Autodesk Inventor part; units mm, degrees
(part 3 of 5)
  line L374 (16.7292, 18.0861) -> (16.8663, 18.4528)
  line L375 (16.8663, 18.4528) -> (16.7213, 18.5673)
  arc A972 (16.7213, 18.5673) -> (16.5062, 18.7273) centre (13.8338, 14.9109) ccw
  arc A973 (16.5062, 18.7273) -> (16.4174, 18.7432) centre (16.4446, 18.6392) ccw
  arc A974 (16.4174, 18.7432) -> (16.3499, 18.6856) centre (16.4431, 18.6448) ccw
  arc A975 (16.3499, 18.6856) -> (16.2535, 18.445) centre (20.1386, 17.0284) ccw
  arc A976 (7.6941, 18.0877) -> (7.7913, 18.19) centre (6.7179, 19.1135) ccw
  arc A977 (7.5704, 17.9771) -> (7.6941, 18.0877) centre (5.8408, 20.0352) ccw
  arc A978 (7.4412, 17.8752) -> (7.5704, 17.9771) centre (5.8587, 20.0139) ccw
  arc A979 (7.3271, 17.7998) -> (7.4412, 17.8752) centre (6.68, 18.9039) ccw
  arc A980 (7.3271, 17.7998) -> (7.1576, 17.6869) centre (8.2213, 16.2738) ccw
  arc A981 (7.1576, 17.6869) -> (7.1147, 17.6052) centre (7.2224, 17.6008) ccw
  arc A982 (7.1147, 17.6052) -> (7.1453, 17.5068) centre (7.2684, 17.599) ccw
  arc A983 (7.1453, 17.5068) -> (7.307, 17.3046) centre (10.3922, 19.9382) ccw
  arc A984 (7.307, 17.3046) -> (7.3807, 17.2275) centre (8.0311, 17.9227) ccw
  arc A985 (7.3807, 17.2275) -> (7.4351, 17.1973) centre (7.468, 17.3209) ccw
  arc A986 (7.4351, 17.1973) -> (7.4946, 17.1979) centre (7.4638, 17.3048) ccw
  arc A987 (7.4946, 17.1979) -> (7.5838, 17.2309) centre (7.3149, 17.821) ccw
  arc A988 (7.5838, 17.2309) -> (7.7872, 17.3447) centre (6.9978, 18.5171) ccw
  arc A989 (7.7872, 17.3447) -> (7.9869, 17.499) centre (6.7051, 18.9518) ccw
  arc A990 (7.9869, 17.499) -> (8.1701, 17.6827) centre (6.6366, 19.0294) ccw
  arc A991 (8.1701, 17.6827) -> (8.3244, 17.8844) centre (6.7621, 18.9192) ccw
  arc A992 (8.3244, 17.8844) -> (8.3941, 17.9924) centre (3.8751, 20.8314) ccw
  arc A993 (8.3941, 17.9924) -> (8.4528, 18.0896) centre (5.6287, 19.7297) ccw
  arc A994 (8.4528, 18.0896) -> (8.4998, 18.1724) centre (4.4364, 20.4221) ccw
  arc A995 (8.4998, 18.1724) -> (8.5063, 18.1976) centre (8.4543, 18.1976) ccw
  arc A996 (8.5063, 18.1976) -> (8.4823, 18.2379) centre (8.4603, 18.1976) ccw
  arc A997 (8.4823, 18.2379) -> (8.2984, 18.3345) centre (5.3457, 12.4849) ccw
  arc A998 (8.2984, 18.3345) -> (8.1156, 18.4216) centre (6.279, 14.3339) ccw
  arc A999 (8.1156, 18.4216) -> (8.0392, 18.4333) centre (8.0563, 18.2894) ccw
  arc A1000 (8.0392, 18.4333) -> (8.014, 18.4217) centre (8.0445, 18.3884) ccw
  arc A1001 (8.014, 18.4217) -> (7.9487, 18.3598) centre (9.8459, 16.4267) ccw
  arc A1002 (7.9487, 18.3598) -> (7.873, 18.2817) centre (9.4826, 16.7968) ccw
  arc A1003 (7.873, 18.2817) -> (7.7913, 18.19) centre (10.4757, 15.8807) ccw
  line L376 (9.6608, 18.2942) -> (9.4652, 18.1559)
  line L377 (9.4652, 18.1559) -> (9.5952, 17.9907)
  arc A1004 (9.5952, 17.9907) -> (9.6704, 17.9062) centre (10.3274, 18.5667) ccw
  arc A1005 (9.6704, 17.9062) -> (9.8032, 17.7781) centre (13.9276, 22.186) ccw
  arc A1006 (9.8032, 17.7781) -> (9.9598, 17.6361) centre (14.449, 22.7432) ccw
  arc A1007 (9.9598, 17.6361) -> (10.1207, 17.499) centre (14.4559, 22.751) ccw
  line L378 (10.1207, 17.499) -> (10.5163, 17.1725)
  line L379 (10.5163, 17.1725) -> (10.6542, 17.3404)
  arc A1008 (10.6542, 17.3404) -> (10.8211, 17.5537) centre (6.2502, 20.9578) ccw
  arc A1009 (10.8211, 17.5537) -> (10.8643, 17.6563) centre (10.634, 17.693) ccw
  arc A1010 (10.8643, 17.6563) -> (10.8379, 17.7313) centre (10.7819, 17.6694) ccw
  arc A1011 (10.8379, 17.7313) -> (10.7285, 17.8072) centre (10.4913, 17.3486) ccw
  arc A1012 (10.6375, 17.8607) -> (10.7285, 17.8072) centre (11.1778, 18.6761) ccw
  arc A1013 (10.5045, 17.952) -> (10.6375, 17.8607) centre (13.4185, 22.0579) ccw
  arc A1014 (10.358, 18.0595) -> (10.5045, 17.952) centre (13.7855, 22.575) ccw
  arc A1015 (10.2183, 18.1693) -> (10.358, 18.0595) centre (13.4932, 22.1899) ccw
  arc A1016 (10.2183, 18.1693) -> (10.0905, 18.2723) centre (0.619, 6.3839) ccw
  arc A1017 (10.0905, 18.2723) -> (9.9804, 18.3585) centre (5.0648, 11.9641) ccw
  arc A1018 (9.9804, 18.3585) -> (9.8833, 18.4328) centre (-8.8499, -6.1368) ccw
  arc A1019 (9.8833, 18.4328) -> (9.8721, 18.4355) centre (9.8747, 18.4215) ccw
  arc A1020 (9.8721, 18.4355) -> (9.8612, 18.431) centre (9.8776, 18.4062) ccw
  arc A1021 (9.8612, 18.431) -> (9.8035, 18.3928) centre (16.1792, 8.8513) ccw
  arc A1022 (9.8035, 18.3928) -> (9.7368, 18.3474) centre (12.5971, 14.212) ccw
  arc A1023 (9.7368, 18.3474) -> (9.6608, 18.2942) centre (14.7573, 11.0889) ccw
  arc A1024 (3.6477, 16.3116) -> (3.7063, 16.3393) centre (3.5663, 16.5594) ccw
  arc A1025 (3.5105, 16.2688) -> (3.6477, 16.3116) centre (2.1461, 20.885) ccw
  arc A1026 (3.3452, 16.2231) -> (3.5105, 16.2688) centre (2.1289, 20.9431) ccw
  arc A1027 (3.1663, 16.1797) -> (3.3452, 16.2231) centre (1.7336, 22.4773) ccw
  arc A1028 (3.1663, 16.1797) -> (2.9905, 16.1377) centre (4.9716, 8.2444) ccw
  arc A1029 (2.9905, 16.1377) -> (2.8348, 16.096) centre (4.2449, 11.1399) ccw
  arc A1030 (2.8348, 16.096) -> (2.7056, 16.0578) centre (4.7069, 9.5159) ccw
  arc A1031 (2.7056, 16.0578) -> (2.6699, 16.0385) centre (2.7354, 15.9603) ccw
  arc A1032 (2.6699, 16.0385) -> (2.6575, 16.01) centre (2.6923, 16.0117) ccw
  arc A1033 (2.6575, 16.01) -> (2.6651, 15.9443) centre (3.1615, 16.0349) ccw
  arc A1034 (2.6651, 15.9443) -> (2.6855, 15.8622) centre (3.3193, 16.0638) ccw
  arc A1035 (2.6855, 15.8622) -> (2.7185, 15.7722) centre (3.7253, 16.1929) ccw
  arc A1036 (2.7185, 15.7722) -> (2.779, 15.6418) centre (4.4501, 16.4957) ccw
  arc A1037 (2.779, 15.6418) -> (2.8266, 15.5869) centre (2.9144, 15.711) ccw
  arc A1038 (2.8266, 15.5869) -> (2.8873, 15.5685) centre (2.8844, 15.6686) ccw
  arc A1039 (2.8873, 15.5685) -> (2.9899, 15.5801) centre (2.8701, 16.1793) ccw
  arc A1040 (3.0973, 15.5961) -> (2.9899, 15.5801) centre (3.2041, 14.5091) ccw
  arc A1041 (3.1411, 15.5806) -> (3.0973, 15.5961) centre (3.1027, 15.5415) ccw
  arc A1042 (3.1621, 15.535) -> (3.1411, 15.5806) centre (3.0918, 15.5304) ccw
  arc A1043 (3.1663, 15.4069) -> (3.1621, 15.535) centre (1.2223, 15.4069) ccw
  arc A1044 (3.1599, 15.2756) -> (3.1663, 15.4069) centre (1.8203, 15.4069) ccw
  arc A1045 (3.1319, 15.225) -> (3.1599, 15.2756) centre (3.0873, 15.2827) ccw
  arc A1046 (3.0711, 15.2026) -> (3.1319, 15.225) centre (3.0659, 15.3104) ccw
  arc A1047 (2.8963, 15.1984) -> (3.0711, 15.2026) centre (2.8963, 18.8358) ccw
  line L380 (2.8963, 15.1984) -> (2.6263, 15.1984)
  line L381 (2.6263, 15.1984) -> (2.6263, 14.9284)
  line L382 (2.6263, 14.9284) -> (2.6263, 14.6584)
  line L383 (2.6263, 14.6584) -> (2.8663, 14.6584)
  arc A1048 (2.9628, 14.6537) -> (2.8663, 14.6584) centre (2.8663, 13.664) ccw
  arc A1049 (3.0393, 14.6391) -> (2.9628, 14.6537) centre (2.9216, 14.2311) ccw
  arc A1050 (3.0903, 14.6171) -> (3.0393, 14.6391) centre (2.978, 14.4266) ccw
  arc A1051 (3.1063, 14.5892) -> (3.0903, 14.6171) centre (3.0739, 14.5892) ccw
  arc A1052 (3.0798, 14.4829) -> (3.1063, 14.5892) centre (2.8798, 14.5892) ccw
  arc A1053 (2.8943, 14.1424) -> (3.0798, 14.4829) centre (-13.1245, 23.093) ccw
  arc A1054 (2.7016, 13.806) -> (2.8943, 14.1424) centre (-13.0788, 23.0674) ccw
  arc A1055 (2.6248, 13.7275) -> (2.7016, 13.806) centre (2.505, 13.9214) ccw
  arc A1056 (2.6248, 13.7275) -> (2.5806, 13.6708) centre (2.6792, 13.6395) ccw
  arc A1057 (2.5806, 13.6708) -> (2.5735, 13.586) centre (2.7631, 13.6128) ccw
  arc A1058 (2.5735, 13.586) -> (2.607, 13.4562) centre (3.1681, 13.6701) ccw
  arc A1059 (2.607, 13.4562) -> (2.6927, 13.2479) centre (6.6369, 14.9926) ccw
  line L384 (2.6927, 13.2479) -> (2.8191, 12.9621)
  line L385 (2.8191, 12.9621) -> (2.9917, 13.2553)
  line L386 (2.9917, 13.2553) -> (3.1642, 13.5484)
  line L387 (3.1642, 13.5484) -> (3.1653, 12.9634)
  line L388 (3.1653, 12.9634) -> (3.1663, 12.3784)
  line L389 (3.1663, 12.3784) -> (3.4663, 12.3784)
  line L390 (3.4663, 12.3784) -> (3.7663, 12.3784)
  line L391 (3.7663, 12.3784) -> (3.7663, 13.0157)
  arc A1060 (3.7687, 13.3861) -> (3.7663, 13.0157) centre (31.5356, 13.0157) ccw
  arc A1061 (3.7816, 13.5332) -> (3.7687, 13.3861) centre (4.767, 13.3728) ccw
  arc A1062 (3.812, 13.5798) -> (3.7816, 13.5332) centre (3.8496, 13.5222) ccw
  arc A1063 (3.8577, 13.5772) -> (3.812, 13.5798) centre (3.8331, 13.5475) ccw
  arc A1064 (3.8577, 13.5772) -> (3.9268, 13.5287) centre (4.1934, 13.9816) ccw
  arc A1065 (3.9268, 13.5287) -> (3.9645, 13.531) centre (3.9439, 13.5577) ccw
  arc A1066 (3.9645, 13.531) -> (3.9959, 13.5732) centre (3.9045, 13.6086) ccw
  arc A1067 (3.9959, 13.5732) -> (4.0533, 13.7284) centre (-1.0766, 15.5375) ccw
  arc A1068 (4.0815, 13.7454) -> (4.0533, 13.7284) centre (4.0777, 13.7198) ccw
  arc A1069 (4.1052, 13.721) -> (4.0815, 13.7454) centre (4.0774, 13.7178) ccw
  arc A1070 (4.1169, 13.5457) -> (4.1052, 13.721) centre (2.3407, 13.5153) ccw
  arc A1071 (4.1215, 13.1434) -> (4.1169, 13.5457) centre (-32.6788, 12.9155) ccw
  line L392 (4.1215, 13.1434) -> (4.1263, 12.3784)
  line L393 (4.1263, 12.3784) -> (4.4263, 12.3784)
  line L394 (4.4263, 12.3784) -> (4.7263, 12.3784)
  line L395 (4.7263, 12.3784) -> (4.7263, 13.4884)
  line L396 (4.7263, 13.4884) -> (4.7263, 14.5984)
  line L397 (4.7263, 14.5984) -> (4.4297, 14.5984)
  line L398 (4.4297, 14.5984) -> (4.1332, 14.5984)
  line L399 (4.1332, 14.5984) -> (4.1147, 14.3468)
  line L400 (4.1147, 14.3468) -> (4.0963, 14.0952)
  line L401 (4.0963, 14.0952) -> (3.9347, 14.3403)
  arc A1072 (3.8326, 14.5081) -> (3.9347, 14.3403) centre (6.2209, 15.8471) ccw
  arc A1073 (3.813, 14.595) -> (3.8326, 14.5081) centre (3.9687, 14.5844) ccw
  arc A1074 (3.8508, 14.6426) -> (3.813, 14.595) centre (3.8665, 14.5913) ccw
  arc A1075 (3.9563, 14.6584) -> (3.8508, 14.6426) centre (3.9563, 14.2981) ccw
  arc A1076 (3.9563, 14.6584) -> (4.0114, 14.6724) centre (3.9563, 14.7736) ccw
  arc A1077 (4.0114, 14.6724) -> (4.0452, 14.7102) centre (3.9753, 14.7387) ccw
  arc A1078 (4.0452, 14.7102) -> (4.0621, 14.7849) centre (3.8283, 14.7986) ccw
  arc A1079 (4.0621, 14.7849) -> (4.0663, 14.9284) centre (1.6148, 14.9284) ccw
  arc A1080 (4.0663, 14.9284) -> (4.0622, 15.0892) centre (0.8993, 14.9284) ccw
  arc A1081 (4.0622, 15.0892) -> (4.0429, 15.1564) centre (3.9078, 15.0813) ccw
  arc A1082 (4.0429, 15.1564) -> (4.0007, 15.1885) centre (3.9854, 15.1244) ccw
  arc A1083 (4.0007, 15.1885) -> (3.9163, 15.1984) centre (3.9163, 14.835) ccw
  arc A1084 (3.8312, 15.209) -> (3.9163, 15.1984) centre (3.9163, 15.5439) ccw
  arc A1085 (3.7889, 15.2428) -> (3.8312, 15.209) centre (3.8474, 15.2726) ccw
  arc A1086 (3.7701, 15.3144) -> (3.7889, 15.2428) centre (3.9439, 15.3218) ccw
  arc A1087 (3.7663, 15.4925) -> (3.7701, 15.3144) centre (7.9201, 15.4925) ccw
  arc A1088 (3.7714, 15.6685) -> (3.7663, 15.4925) centre (6.7776, 15.4925) ccw
  arc A1089 (3.7936, 15.7512) -> (3.7714, 15.6685) centre (3.9835, 15.6561) ccw
  arc A1090 (3.8431, 15.8031) -> (3.7936, 15.7512) centre (3.9028, 15.6965) ccw
  arc A1091 (3.9448, 15.8489) -> (3.8431, 15.8031) centre (4.1545, 15.2472) ccw
  arc A1092 (4.05, 15.8781) -> (3.9448, 15.8489) centre (4.2234, 15.0497) ccw
  arc A1093 (4.1141, 15.8736) -> (4.05, 15.8781) centre (4.0741, 15.7629) ccw
  arc A1094 (4.1695, 15.8357) -> (4.1141, 15.8736) centre (4.0685, 15.7473) ccw
  arc A1095 (4.2448, 15.7405) -> (4.1695, 15.8357) centre (3.2556, 15.0361) ccw
  arc A1096 (4.2448, 15.7405) -> (4.3218, 15.647) centre (4.9481, 16.2412) ccw
  arc A1097 (4.3218, 15.647) -> (4.3884, 15.6028) centre (4.4513, 15.7699) ccw
  arc A1098 (4.3884, 15.6028) -> (4.4736, 15.5884) centre (4.4678, 15.8136) ccw
  arc A1099 (4.4736, 15.5884) -> (4.6213, 15.5987) centre (4.4293, 17.2943) ccw
  arc A1100 (4.6213, 15.5987) -> (4.9936, 15.6499) centre (3.739, 23.3885) ccw
  arc A1101 (4.9936, 15.6499) -> (5.4376, 15.7283) centre (2.4091, 31.5923) ccw
  arc A1102 (5.4376, 15.7283) -> (5.8624, 15.8155) centre (2.4855, 31.1919) ccw
  arc A1103 (5.8624, 15.8155) -> (6.1634, 15.8931) centre (4.9424, 20.0048) ccw
  line L402 (6.1634, 15.8931) -> (6.4843, 15.9884)
  line L403 (6.4843, 15.9884) -> (6.2757, 16.197)
  line L404 (6.2757, 16.197) -> (6.0672, 16.4055)
  line L405 (6.0672, 16.4055) -> (5.5926, 16.2812)
  arc A1104 (5.3759, 16.2309) -> (5.5926, 16.2812) centre (4.5848, 20.129) ccw
  arc A1105 (5.1154, 16.1825) -> (5.3759, 16.2309) centre (3.7927, 24.032) ccw
  arc A1106 (4.8539, 16.1429) -> (5.1154, 16.1825) centre (3.7959, 24.0132) ccw
  arc A1107 (4.6343, 16.1197) -> (4.8539, 16.1429) centre (4.3369, 19.9889) ccw
  arc A1108 (4.3228, 16.0993) -> (4.6343, 16.1197) centre (3.5643, 30.0399) ccw
  arc A1109 (4.2008, 16.1084) -> (4.3228, 16.0993) centre (4.2969, 16.5759) ccw
  arc A1110 (4.1235, 16.1488) -> (4.2008, 16.1084) centre (4.2327, 16.2636) ccw
  arc A1111 (4.047, 16.2405) -> (4.1235, 16.1488) centre (4.4815, 16.5252) ccw
  arc A1112 (4.047, 16.2405) -> (3.9666, 16.3415) centre (3.4613, 15.8567) ccw
  arc A1113 (3.9666, 16.3415) -> (3.8904, 16.3876) centre (3.8425, 16.2224) ccw
  arc A1114 (3.8904, 16.3876) -> (3.8073, 16.3865) centre (3.8506, 16.2503) ccw
  arc A1115 (3.8073, 16.3865) -> (3.7063, 16.3393) centre (3.9382, 15.9746) ccw
  arc A1116 (8.0014, 16.2036) -> (8.0263, 16.2484) centre (7.9734, 16.2484) ccw
  arc A1117 (7.9313, 16.1762) -> (8.0014, 16.2036) centre (7.8939, 16.3757) ccw
  arc A1118 (7.7978, 16.1619) -> (7.9313, 16.1762) centre (7.7739, 17.0157) ccw
  arc A1119 (7.5463, 16.1584) -> (7.7978, 16.1619) centre (7.5463, 25.1492) ccw
  line L406 (7.5463, 16.1584) -> (7.0663, 16.1584)
  line L407 (7.0663, 16.1584) -> (7.0663, 15.9184)
  line L408 (7.0663, 15.9184) -> (7.0663, 15.6784)
  line L409 (7.0663, 15.6784) -> (7.5463, 15.6784)
  arc A1120 (7.7978, 15.6749) -> (7.5463, 15.6784) centre (7.5463, 6.6876) ccw
  arc A1121 (7.9313, 15.6606) -> (7.7978, 15.6749) centre (7.7739, 14.8211) ccw
  arc A1122 (8.0014, 15.6332) -> (7.9313, 15.6606) centre (7.8939, 15.4611) ccw
  arc A1123 (8.0263, 15.5884) -> (8.0014, 15.6332) centre (7.9734, 15.5884) ccw
  arc A1124 (8.0142, 15.5495) -> (8.0263, 15.5884) centre (7.9577, 15.5884) ccw
  arc A1125 (7.9813, 15.5209) -> (8.0142, 15.5495) centre (7.9422, 15.5991) ccw
  arc A1126 (7.9256, 15.5037) -> (7.9813, 15.5209) centre (7.9018, 15.6799) ccw
  arc A1127 (7.8463, 15.4984) -> (7.9256, 15.5037) centre (7.8463, 16.0905) ccw
  arc A1128 (7.8463, 15.4984) -> (7.767, 15.4931) centre (7.8463, 14.9063) ccw
  arc A1129 (7.767, 15.4931) -> (7.7113, 15.4759) centre (7.7908, 15.3169) ccw
  arc A1130 (7.7113, 15.4759) -> (7.6784, 15.4473) centre (7.7504, 15.3977) ccw
  arc A1131 (7.6784, 15.4473) -> (7.6663, 15.4084) centre (7.7349, 15.4084) ccw
  arc A1132 (7.6486, 15.366) -> (7.6663, 15.4084) centre (7.6066, 15.4084) ccw
  arc A1133 (7.6013, 15.3379) -> (7.6486, 15.366) centre (7.5686, 15.4468) ccw
  arc A1134 (7.5139, 15.3226) -> (7.6013, 15.3379) centre (7.4926, 15.7) ccw
  arc A1135 (7.3663, 15.3184) -> (7.5139, 15.3226) centre (7.3663, 17.9435) ccw
  line L410 (7.3663, 15.3184) -> (7.0663, 15.3184)
  line L411 (7.0663, 15.3184) -> (7.0663, 15.0784)
  line L412 (7.0663, 15.0784) -> (7.0663, 14.8384)
  line L413 (7.0663, 14.8384) -> (7.3663, 14.8384)
  line L414 (7.3663, 14.8384) -> (7.6663, 14.8384)
  line L415 (7.6663, 14.8384) -> (7.6663, 14.3584)
  line L416 (7.6663, 14.3584) -> (7.6663, 13.8784)
  line L417 (7.6663, 13.8784) -> (8.1763, 13.8784)
  arc A1136 (8.3814, 13.8744) -> (8.1763, 13.8784) centre (8.1763, 8.6641) ccw
  arc A1137 (8.5438, 13.8616) -> (8.3814, 13.8744) centre (8.299, 11.781) ccw
  arc A1138 (8.6654, 13.8434) -> (8.5438, 13.8616) centre (8.3148, 11.9152) ccw
  arc A1139 (8.6863, 13.8184) -> (8.6654, 13.8434) centre (8.6608, 13.8184) ccw
  arc A1140 (8.6624, 13.7919) -> (8.6863, 13.8184) centre (8.6596, 13.8184) ccw
  arc A1141 (8.4688, 13.7745) -> (8.6624, 13.7919) centre (8.0091, 19.9801) ccw
  arc A1142 (8.214, 13.7622) -> (8.4688, 13.7745) centre (8.102, 18.7256) ccw
  arc A1143 (7.8763, 13.7584) -> (8.214, 13.7622) centre (7.8763, 28.7312) ccw
  line L418 (7.8763, 13.7584) -> (7.0663, 13.7584)
  line L419 (7.0663, 13.7584) -> (7.0663, 13.5184)
  line L420 (7.0663, 13.5184) -> (7.0663, 13.2784)
  line L421 (7.0663, 13.2784) -> (7.5913, 13.2759)
  line L422 (7.5913, 13.2759) -> (8.1163, 13.2734)
  line L423 (8.1163, 13.2734) -> (7.9063, 13.159)
  arc A1144 (7.8035, 13.11) -> (7.9063, 13.159) centre (7.3969, 14.0942) ccw
  arc A1145 (7.6654, 13.0569) -> (7.8035, 13.11) centre (6.6636, 15.8691) ccw
  arc A1146 (7.5172, 13.0081) -> (7.6654, 13.0569) centre (6.5956, 16.0598) ccw
  arc A1147 (7.3813, 12.972) -> (7.5172, 13.0081) centre (6.9066, 15.03) ccw
  arc A1148 (7.3813, 12.972) -> (7.2605, 12.9425) centre (8.5241, 8.0169) ccw
  arc A1149 (7.2605, 12.9425) -> (7.1588, 12.9143) centre (7.9205, 10.3697) ccw
  arc A1150 (7.1588, 12.9143) -> (7.074, 12.8881) centre (8.7518, 7.5926) ccw
  arc A1151 (7.074, 12.8881) -> (7.0663, 12.8777) centre (7.0773, 12.8777) ccw
  arc A1152 (7.0663, 12.8777) -> (7.0702, 12.8627) centre (7.0966, 12.8777) ccw
  arc A1153 (7.0702, 12.8627) -> (7.1107, 12.792) centre (14.3749, 16.9978) ccw
  arc A1154 (7.1107, 12.792) -> (7.1596, 12.7098) centre (10.6995, 14.8698) ccw
  arc A1155 (7.1596, 12.7098) -> (7.2176, 12.6164) centre (13.3252, 16.472) ccw
  arc A1156 (7.2176, 12.6164) -> (7.3075, 12.4843) centre (9.1632, 13.8446) ccw
  arc A1157 (7.3075, 12.4843) -> (7.371, 12.4246) centre (7.4997, 12.6252) ccw
  arc A1158 (7.371, 12.4246) -> (7.4384, 12.4043) centre (7.4403, 12.5327) ccw
  arc A1159 (7.4384, 12.4043) -> (7.5326, 12.4142) centre (7.4444, 12.7994) ccw
  arc A1160 (7.5326, 12.4142) -> (7.7412, 12.4788) centre (7.2096, 13.8264) ccw
  arc A1161 (7.7412, 12.4788) -> (8.0301, 12.6017) centre (5.5636, 17.9992) ccw
  arc A1162 (8.0301, 12.6017) -> (8.3142, 12.7408) centre (5.5696, 17.9861) ccw
  arc A1163 (8.3142, 12.7408) -> (8.5093, 12.8605) centre (7.5371, 14.2258) ccw
  line L424 (8.5093, 12.8605) -> (8.6863, 12.9866)
  line L425 (8.6863, 12.9866) -> (8.6863, 12.6825)
  line L426 (8.6863, 12.6825) -> (8.6863, 12.3784)
  line L427 (8.6863, 12.3784) -> (8.9863, 12.3784)
  line L428 (8.9863, 12.3784) -> (9.2863, 12.3784)
  line L429 (9.2863, 12.3784) -> (9.2863, 12.6784)
  arc A1164 (9.2889, 12.7934) -> (9.2863, 12.6784) centre (11.8588, 12.6784) ccw
  arc A1165 (9.2968, 12.8903) -> (9.2889, 12.7934) centre (10.6038, 12.7346) ccw
  arc A1166 (9.3078, 12.9665) -> (9.2968, 12.8903) centre (10.7802, 12.7136) ccw
  arc A1167 (9.322, 12.9784) -> (9.3078, 12.9665) centre (9.322, 12.964) ccw
  arc A1168 (9.3436, 12.9731) -> (9.322, 12.9784) centre (9.322, 12.9321) ccw
  arc A1169 (9.394, 12.9452) -> (9.3436, 12.9731) centre (8.6908, 11.7331) ccw
  arc A1170 (9.4534, 12.9086) -> (9.394, 12.9452) centre (8.7299, 11.8005) ccw
  arc A1171 (9.517, 12.8653) -> (9.4534, 12.9086) centre (8.3809, 11.266) ccw
  arc A1172 (9.517, 12.8653) -> (9.7267, 12.7415) centre (10.3528, 14.0417) ccw
  arc A1173 (9.7267, 12.7415) -> (10.0544, 12.5947) centre (12.5439, 18.5921) ccw
  arc A1174 (10.0544, 12.5947) -> (10.3832, 12.4669) centre (13.037, 19.7799) ccw
  arc A1175 (10.3832, 12.4669) -> (10.5454, 12.4384) centre (10.5454, 12.9139) ccw
  arc A1176 (10.5454, 12.4384) -> (10.6465, 12.4779) centre (10.5454, 12.5874) ccw
  arc A1177 (10.6465, 12.4779) -> (10.7756, 12.6185) centre (9.8563, 13.3335) ccw
  arc A1178 (10.7756, 12.6185) -> (10.8795, 12.7772) centre (9.8531, 13.336) ccw
  arc A1179 (10.8795, 12.7772) -> (10.8888, 12.88) centre (10.7653, 12.8394) ccw
  arc A1180 (10.8888, 12.88) -> (10.8656, 12.906) centre (10.8474, 12.8664) ccw
  arc A1181 (10.8656, 12.906) -> (10.7365, 12.963) centre (8.7774, 8.3472) ccw
  arc A1182 (10.7365, 12.963) -> (10.5784, 13.0256) centre (9.3779, 9.7622) ccw
  arc A1183 (10.5784, 13.0256) -> (10.3941, 13.09) centre (8.4963, 7.3655) ccw
  line L430 (10.3941, 13.09) -> (9.9163, 13.2484)
  line L431 (9.9163, 13.2484) -> (10.4113, 13.2658)
  line L432 (10.4113, 13.2658) -> (10.9063, 13.2833)
  line L433 (10.9063, 13.2833) -> (10.9063, 13.5208)
  line L434 (10.9063, 13.5208) -> (10.9063, 13.7584)
  line L435 (10.9063, 13.7584) -> (10.1298, 13.7584)
  arc A1184 (9.8171, 13.7625) -> (10.1298, 13.7584) centre (10.1298, 25.6917) ccw
  arc A1185 (9.5613, 13.7753) -> (9.8171, 13.7625) centre (9.9586, 19.1627) ccw
  arc A1186 (9.3565, 13.7932) -> (9.5613, 13.7753) centre (10.1116, 21.2371) ccw
  arc A1187 (9.3163, 13.8184) -> (9.3565, 13.7932) centre (9.362, 13.8466) ccw
  arc A1188 (9.3285, 13.8452) -> (9.3163, 13.8184) centre (9.3314, 13.8277) ccw
  arc A1189 (9.4679, 13.8629) -> (9.3285, 13.8452) centre (9.6507, 11.8624) ccw
  arc A1190 (9.6754, 13.8748) -> (9.4679, 13.8629) centre (9.7492, 10.7855) ccw
  arc A1191 (9.9727, 13.8784) -> (9.6754, 13.8748) centre (9.9727, 1.4213) ccw
  line L436 (9.9727, 13.8784) -> (10.6663, 13.8784)
  line L437 (10.6663, 13.8784) -> (10.6663, 14.1184)
  line L438 (10.6663, 14.1184) -> (10.6663, 14.3584)
  line L439 (10.6663, 14.3584) -> (9.4663, 14.3584)
  line L440 (9.4663, 14.3584) -> (8.2663, 14.3584)
  line L441 (8.2663, 14.3584) -> (8.2663, 14.5984)
  line L442 (8.2663, 14.5984) -> (8.2663, 14.8384)
  line L443 (8.2663, 14.8384) -> (8.5063, 14.8384)
  arc A1192 (8.6575, 14.8336) -> (8.5063, 14.8384) centre (8.5063, 12.4478) ccw
  arc A1193 (8.7141, 14.8103) -> (8.6575, 14.8336) centre (8.6515, 14.7387) ccw
  arc A1194 (8.7403, 14.7589) -> (8.7141, 14.8103) centre (8.663, 14.7518) ccw
  arc A1195 (8.7463, 14.6284) -> (8.7403, 14.7589) centre (7.3117, 14.6284) ccw
  line L444 (8.7463, 14.6284) -> (8.7463, 14.4184)
  line L445 (8.7463, 14.4184) -> (9.4963, 14.4184)
  line L446 (9.4963, 14.4184) -> (10.2463, 14.4184)
  line L447 (10.2463, 14.4184) -> (10.2463, 14.6284)
  line L448 (10.2463, 14.6284) -> (10.2463, 14.8384)
  line L449 (10.2463, 14.8384) -> (10.5763, 14.8384)
  line L450 (10.5763, 14.8384) -> (10.9063, 14.8384)
  line L451 (10.9063, 14.8384) -> (10.9063, 15.0784)
  line L452 (10.9063, 15.0784) -> (10.9063, 15.3184)
  line L453 (10.9063, 15.3184) -> (10.5763, 15.3184)
  arc A1196 (10.4114, 15.3224) -> (10.5763, 15.3184) centre (10.5763, 18.7208) ccw
  arc A1197 (10.3163, 15.3375) -> (10.4114, 15.3224) centre (10.4329, 15.765) ccw
  arc A1198 (10.2653, 15.3655) -> (10.3163, 15.3375) centre (10.3491, 15.4577) ccw
  arc A1199 (10.2463, 15.4084) -> (10.2653, 15.3655) centre (10.3043, 15.4084) ccw
  arc A1200 (10.2463, 15.4084) -> (10.2356, 15.4456) centre (10.1761, 15.4084) ccw
  arc A1201 (10.2356, 15.4456) -> (10.2063, 15.4744) centre (10.161, 15.399) ccw
  arc A1202 (10.2063, 15.4744) -> (10.1589, 15.4925) centre (10.1317, 15.3501) ccw
  arc A1203 (10.1589, 15.4925) -> (10.0963, 15.4984) centre (10.0963, 15.1643) ccw
  arc A1204 (10.0337, 15.5043) -> (10.0963, 15.4984) centre (10.0963, 15.8325) ccw
  arc A1205 (9.9863, 15.5224) -> (10.0337, 15.5043) centre (10.0608, 15.6466) ccw
  arc A1206 (9.9569, 15.5512) -> (9.9863, 15.5224) centre (10.0315, 15.5978) ccw
  arc A1207 (9.9463, 15.5884) -> (9.9569, 15.5512) centre (10.0165, 15.5884) ccw
  arc A1208 (9.9711, 15.6332) -> (9.9463, 15.5884) centre (9.9991, 15.5884) ccw
  arc A1209 (10.0413, 15.6606) -> (9.9711, 15.6332) centre (10.0787, 15.4611) ccw
  arc A1210 (10.1748, 15.6749) -> (10.0413, 15.6606) centre (10.1987, 14.8211) ccw
  arc A1211 (10.4263, 15.6784) -> (10.1748, 15.6749) centre (10.4263, 6.6876) ccw
  line L454 (10.4263, 15.6784) -> (10.9063, 15.6784)
  line L455 (10.9063, 15.6784) -> (10.9063, 15.9184)
  line L456 (10.9063, 15.9184) -> (10.9063, 16.1584)
  line L457 (10.9063, 16.1584) -> (10.4263, 16.1584)
  arc A1212 (10.1748, 16.1619) -> (10.4263, 16.1584) centre (10.4263, 25.1492) ccw
  arc A1213 (10.0413, 16.1762) -> (10.1748, 16.1619) centre (10.1987, 17.0157) ccw
  arc A1214 (9.9711, 16.2036) -> (10.0413, 16.1762) centre (10.0787, 16.3757) ccw
  arc A1215 (9.9463, 16.2484) -> (9.9711, 16.2036) centre (9.9991, 16.2484) ccw
  arc A1216 (9.9463, 16.2484) -> (9.9286, 16.2908) centre (9.8866, 16.2484) ccw
  arc A1217 (9.9286, 16.2908) -> (9.8813, 16.3189) centre (9.8486, 16.21) ccw
  arc A1218 (9.8813, 16.3189) -> (9.7939, 16.3342) centre (9.7726, 15.9568) ccw
  arc A1219 (9.7939, 16.3342) -> (9.6463, 16.3384) centre (9.6463, 13.7133) ccw
  arc A1220 (9.6463, 16.3384) -> (9.4986, 16.3342) centre (9.6463, 13.7133) ccw
  arc A1221 (9.4986, 16.3342) -> (9.4113, 16.3189) centre (9.5199, 15.9568) ccw
  arc A1222 (9.4113, 16.3189) -> (9.364, 16.2908) centre (9.4439, 16.21) ccw
  arc A1223 (9.364, 16.2908) -> (9.3463, 16.2484) centre (9.406, 16.2484) ccw
  arc A1224 (9.326, 16.205) -> (9.3463, 16.2484) centre (9.2897, 16.2484) ccw
  arc A1225 (9.2713, 16.1771) -> (9.326, 16.205) centre (9.238, 16.3101) ccw
  arc A1226 (9.1684, 16.1623) -> (9.2713, 16.1771) centre (9.1466, 16.6758) ccw
  arc A1227 (8.9863, 16.1584) -> (9.1684, 16.1623) centre (8.9863, 20.4503) ccw
  arc A1228 (8.8041, 16.1623) -> (8.9863, 16.1584) centre (8.9863, 20.4503) ccw
  arc A1229 (8.7013, 16.1771) -> (8.8041, 16.1623) centre (8.8259, 16.6758) ccw
  arc A1230 (8.6465, 16.205) -> (8.7013, 16.1771) centre (8.7345, 16.3101) ccw
  arc A1231 (8.6263, 16.2484) -> (8.6465, 16.205) centre (8.6828, 16.2484) ccw
  arc A1232 (8.6263, 16.2484) -> (8.6086, 16.2908) centre (8.5666, 16.2484) ccw
  arc A1233 (8.6086, 16.2908) -> (8.5613, 16.3189) centre (8.5286, 16.21) ccw
  arc A1234 (8.5613, 16.3189) -> (8.4739, 16.3342) centre (8.4526, 15.9568) ccw
  arc A1235 (8.4739, 16.3342) -> (8.3263, 16.3384) centre (8.3263, 13.7133) ccw
  arc A1236 (8.3263, 16.3384) -> (8.1786, 16.3342) centre (8.3263, 13.7133) ccw
  arc A1237 (8.1786, 16.3342) -> (8.0913, 16.3189) centre (8.1999, 15.9568) ccw
  arc A1238 (8.0913, 16.3189) -> (8.044, 16.2908) centre (8.1239, 16.21) ccw
  arc A1239 (8.044, 16.2908) -> (8.0263, 16.2484) centre (8.086, 16.2484) ccw
  arc A1240 (9.3463, 15.5884) -> (9.3569, 15.5512) centre (9.4165, 15.5884) ccw
  arc A1241 (9.3569, 15.5512) -> (9.3863, 15.5224) centre (9.4315, 15.5978) ccw
  arc A1242 (9.3863, 15.5224) -> (9.4337, 15.5043) centre (9.4608, 15.6466) ccw
  arc A1243 (9.4337, 15.5043) -> (9.4963, 15.4984) centre (9.4963, 15.8325) ccw
  arc A1244 (9.5589, 15.4925) -> (9.4963, 15.4984) centre (9.4963, 15.1643) ccw
  arc A1245 (9.6063, 15.4744) -> (9.5589, 15.4925) centre (9.5317, 15.3501) ccw
  arc A1246 (9.6356, 15.4456) -> (9.6063, 15.4744) centre (9.561, 15.399) ccw
  arc A1247 (9.6463, 15.4084) -> (9.6356, 15.4456) centre (9.5761, 15.4084) ccw
  arc A1248 (9.6342, 15.3695) -> (9.6463, 15.4084) centre (9.5777, 15.4084) ccw
  arc A1249 (9.6013, 15.3409) -> (9.6342, 15.3695) centre (9.5622, 15.4191) ccw
  arc A1250 (9.5456, 15.3237) -> (9.6013, 15.3409) centre (9.5218, 15.4999) ccw
  arc A1251 (9.4663, 15.3184) -> (9.5456, 15.3237) centre (9.4663, 15.9105) ccw
  arc A1252 (9.387, 15.3237) -> (9.4663, 15.3184) centre (9.4663, 15.9105) ccw
  arc A1253 (9.3313, 15.3409) -> (9.387, 15.3237) centre (9.4108, 15.4999) ccw
  arc A1254 (9.2984, 15.3695) -> (9.3313, 15.3409) centre (9.3704, 15.4191) ccw
  arc A1255 (9.2863, 15.4084) -> (9.2984, 15.3695) centre (9.3549, 15.4084) ccw
  arc A1256 (9.2863, 15.4084) -> (9.2699, 15.4502) centre (9.2246, 15.4084) ccw
  arc A1257 (9.2699, 15.4502) -> (9.2263, 15.4784) centre (9.1933, 15.3794) ccw
  arc A1258 (9.2263, 15.4784) -> (9.1467, 15.494) centre (9.1255, 15.176) ccw
  arc A1259 (9.1467, 15.494) -> (9.0163, 15.4984) centre (9.0163, 13.5405) ccw
  arc A1260 (9.0163, 15.4984) -> (8.8858, 15.494) centre (9.0163, 13.5405) ccw
  arc A1261 (8.8858, 15.494) -> (8.8063, 15.4784) centre (8.9071, 15.176) ccw
  arc A1262 (8.8063, 15.4784) -> (8.7626, 15.4502) centre (8.8393, 15.3794) ccw
  arc A1263 (8.7626, 15.4502) -> (8.7463, 15.4084) centre (8.8079, 15.4084) ccw
  arc A1264 (8.7313, 15.3673) -> (8.7463, 15.4084) centre (8.6824, 15.4084) ccw
  arc A1265 (8.6913, 15.339) -> (8.7313, 15.3673) centre (8.6574, 15.4295) ccw
  arc A1266 (8.6196, 15.323) -> (8.6913, 15.339) centre (8.5981, 15.5876) ccw
  arc A1267 (8.5063, 15.3184) -> (8.6196, 15.323) centre (8.5063, 16.7173) ccw
  arc A1268 (8.393, 15.323) -> (8.5063, 15.3184) centre (8.5063, 16.7173) ccw
  arc A1269 (8.3213, 15.339) -> (8.393, 15.323) centre (8.4145, 15.5876) ccw
  arc A1270 (8.2813, 15.3673) -> (8.3213, 15.339) centre (8.3552, 15.4295) ccw
  arc A1271 (8.2663, 15.4084) -> (8.2813, 15.3673) centre (8.3301, 15.4084) ccw
  arc A1272 (8.2784, 15.4473) -> (8.2663, 15.4084) centre (8.3349, 15.4084) ccw
  arc A1273 (8.3113, 15.4759) -> (8.2784, 15.4473) centre (8.3504, 15.3977) ccw
  arc A1274 (8.367, 15.4931) -> (8.3113, 15.4759) centre (8.3908, 15.3169) ccw
  arc A1275 (8.4463, 15.4984) -> (8.367, 15.4931) centre (8.4463, 14.9063) ccw
  arc A1276 (8.4463, 15.4984) -> (8.5256, 15.5037) centre (8.4463, 16.0905) ccw
  arc A1277 (8.5256, 15.5037) -> (8.5813, 15.5209) centre (8.5018, 15.6799) ccw
  arc A1278 (8.5813, 15.5209) -> (8.6142, 15.5495) centre (8.5422, 15.5991) ccw
  arc A1279 (8.6142, 15.5495) -> (8.6263, 15.5884) centre (8.5577, 15.5884) ccw
  arc A1280 (8.6465, 15.6318) -> (8.6263, 15.5884) centre (8.6828, 15.5884) ccw
  arc A1281 (8.7013, 15.6596) -> (8.6465, 15.6318) centre (8.7345, 15.5267) ccw
  arc A1282 (8.8041, 15.6745) -> (8.7013, 15.6596) centre (8.8259, 15.161) ccw
  arc A1283 (8.9863, 15.6784) -> (8.8041, 15.6745) centre (8.9863, 11.3865) ccw
  arc A1284 (9.1684, 15.6745) -> (8.9863, 15.6784) centre (8.9863, 11.3865) ccw
  arc A1285 (9.2713, 15.6596) -> (9.1684, 15.6745) centre (9.1466, 15.161) ccw
  arc A1286 (9.326, 15.6318) -> (9.2713, 15.6596) centre (9.238, 15.5267) ccw
  arc A1287 (9.3463, 15.5884) -> (9.326, 15.6318) centre (9.2897, 15.5884) ccw
  arc A1288 (9.6337, 14.7553) -> (9.6463, 14.7784) centre (9.6189, 14.7784) ccw
  arc A1289 (9.5934, 14.736) -> (9.6337, 14.7553) centre (9.5368, 14.9057) ccw
  arc A1290 (9.5352, 14.7228) -> (9.5934, 14.736) centre (9.4966, 15.0263) ccw
  arc A1291 (9.4663, 14.7184) -> (9.5352, 14.7228) centre (9.4663, 15.2651) ccw
  arc A1292 (9.3973, 14.7228) -> (9.4663, 14.7184) centre (9.4663, 15.2651) ccw
  arc A1293 (9.3392, 14.736) -> (9.3973, 14.7228) centre (9.4359, 15.0263) ccw
  arc A1294 (9.2989, 14.7553) -> (9.3392, 14.736) centre (9.3957, 14.9057) ccw
  arc A1295 (9.2863, 14.7784) -> (9.2989, 14.7553) centre (9.3137, 14.7784) ccw
  arc A1296 (9.2989, 14.8015) -> (9.2863, 14.7784) centre (9.3137, 14.7784) ccw
  arc A1297 (9.3392, 14.8208) -> (9.2989, 14.8015) centre (9.3957, 14.6511) ccw
  arc A1298 (9.3973, 14.834) -> (9.3392, 14.8208) centre (9.4359, 14.5305) ccw
  arc A1299 (9.4663, 14.8384) -> (9.3973, 14.834) centre (9.4663, 14.2917) ccw
  arc A1300 (9.5352, 14.834) -> (9.4663, 14.8384) centre (9.4663, 14.2917) ccw
  arc A1301 (9.5934, 14.8208) -> (9.5352, 14.834) centre (9.4966, 14.5305) ccw
  arc A1302 (9.6337, 14.8015) -> (9.5934, 14.8208) centre (9.5368, 14.6511) ccw
  arc A1303 (9.6463, 14.7784) -> (9.6337, 14.8015) centre (9.6189, 14.7784) ccw
  arc A1304 (18.4063, 16.0684) -> (18.4112, 15.9765) centre (19.2676, 16.0684) ccw
  arc A1305 (18.4112, 15.9765) -> (18.4272, 15.9115) centre (18.6599, 16.0032) ccw
  arc A1306 (18.4272, 15.9115) -> (18.4535, 15.8726) centre (18.5278, 15.9511) ccw
  arc A1307 (18.4535, 15.8726) -> (18.4891, 15.8584) centre (18.4891, 15.9102) ccw
  arc A1308 (18.5652, 15.8266) -> (18.4891, 15.8584) centre (18.4891, 15.7511) ccw
  arc A1309 (18.7744, 15.6084) -> (18.5652, 15.8266) centre (12.0578, 9.3805) ccw
  arc A1310 (18.9752, 15.3841) -> (18.7744, 15.6084) centre (12.466, 9.7589) ccw
  arc A1311 (19.0063, 15.3006) -> (18.9752, 15.3841) centre (18.8785, 15.3006) ccw
  arc A1312 (18.9986, 15.2865) -> (19.0063, 15.3006) centre (18.9895, 15.3006) ccw
  arc A1313 (18.9534, 15.2592) -> (18.9986, 15.2865) centre (18.4772, 16.098) ccw
  arc A1314 (18.8953, 15.229) -> (18.9534, 15.2592) centre (18.5198, 16.0231) ccw
  arc A1315 (18.8263, 15.1984) -> (18.8953, 15.229) centre (18.237, 16.621) ccw
  arc A1316 (18.8263, 15.1984) -> (18.6958, 15.1406) centre (19.9591, 12.4635) ccw
  arc A1317 (18.6958, 15.1406) -> (18.6594, 15.1051) centre (18.729, 15.0701) ccw
  arc A1318 (18.6594, 15.1051) -> (18.6579, 15.0594) centre (18.708, 15.0807) ccw
  arc A1319 (18.6579, 15.0594) -> (18.7059, 14.9591) centre (19.7938, 15.5413) ccw
  arc A1320 (18.7297, 14.8983) -> (18.7059, 14.9591) centre (18.4618, 14.8285) ccw
  arc A1321 (18.7214, 14.8606) -> (18.7297, 14.8983) centre (18.6885, 14.8876) ccw
  arc A1322 (18.681, 14.8335) -> (18.7214, 14.8606) centre (18.6563, 14.9139) ccw
  arc A1323 (18.5816, 14.8074) -> (18.681, 14.8335) centre (18.3096, 16.0458) ccw
  arc A1324 (18.509, 14.7941) -> (18.5816, 14.8074) centre (18.3555, 15.8368) ccw
  arc A1325 (18.443, 14.7876) -> (18.509, 14.7941) centre (18.4087, 15.4753) ccw
  arc A1326 (18.3895, 14.7873) -> (18.443, 14.7876) centre (18.413, 15.3895) ccw
  arc A1327 (18.368, 14.7967) -> (18.3895, 14.7873) centre (18.3908, 14.8196) ccw
  arc A1328 (18.3622, 14.8204) -> (18.368, 14.7967) centre (18.3845, 14.8133) ccw
  arc A1329 (18.3919, 14.9064) -> (18.3622, 14.8204) centre (20.2177, 14.228) ccw
  arc A1330 (18.4346, 15.0104) -> (18.3919, 14.9064) centre (19.9193, 14.3389) ccw
  arc A1331 (18.4911, 15.1282) -> (18.4346, 15.0104) centre (21.1234, 13.7943) ccw
  line L458 (18.4911, 15.1282) -> (18.644, 15.4299)
  line L459 (18.644, 15.4299) -> (18.4316, 15.4999)
  arc A1332 (18.3107, 15.5456) -> (18.4316, 15.4999) centre (18.9136, 16.9604) ccw
  arc A1333 (18.2597, 15.5859) -> (18.3107, 15.5456) centre (18.3592, 15.6592) ccw
  arc A1334 (18.2431, 15.6411) -> (18.2597, 15.5859) centre (18.3286, 15.6367) ccw
  arc A1335 (18.2561, 15.7377) -> (18.2431, 15.6411) centre (18.8345, 15.6107) ccw
  arc A1336 (18.2561, 15.7377) -> (18.2669, 15.8307) centre (17.8032, 15.8372) ccw
  arc A1337 (18.2669, 15.8307) -> (18.2516, 15.8986) centre (18.1181, 15.8328) ccw
  arc A1338 (18.2516, 15.8986) -> (18.2045, 15.9604) centre (18.0701, 15.8092) ccw
  arc A1339 (18.2045, 15.9604) -> (18.1088, 16.0366) centre (17.4503, 15.1117) ccw
  line L460 (18.1088, 16.0366) -> (17.9247, 16.1677)
  line L461 (17.9247, 16.1677) -> (17.5972, 15.8213)
  arc A1340 (17.4683, 15.6921) -> (17.5972, 15.8213) centre (15.1322, 18.1523) ccw
  arc A1341 (17.3522, 15.5914) -> (17.4683, 15.6921) centre (16.2868, 16.9364) ccw
  arc A1342 (17.2564, 15.5212) -> (17.3522, 15.5914) centre (16.357, 16.8477) ccw
  arc A1343 (17.223, 15.5249) -> (17.2564, 15.5212) centre (17.2419, 15.5426) ccw
  arc A1344 (17.2111, 15.546) -> (17.223, 15.5249) centre (17.2601, 15.5596) ccw
  arc A1345 (17.212, 15.568) -> (17.2111, 15.546) centre (17.2457, 15.5556) ccw
  arc A1346 (17.2262, 15.5876) -> (17.212, 15.568) centre (17.2542, 15.5525) ccw
  arc A1347 (17.2513, 15.6016) -> (17.2262, 15.5876) centre (17.2806, 15.5194) ccw
  arc A1348 (17.2513, 15.6016) -> (17.2819, 15.6292) centre (17.2331, 15.6525) ccw
  arc A1349 (17.2819, 15.6292) -> (17.3055, 15.6943) centre (16.9585, 15.7835) ccw
  arc A1350 (17.3055, 15.6943) -> (17.3212, 15.7843) centre (16.7462, 15.8381) ccw
  arc A1351 (17.3212, 15.7843) -> (17.3263, 15.8934) centre (16.1551, 15.8934) ccw
  line L462 (17.3263, 15.8934) -> (17.3263, 16.1584)
  line L463 (17.3263, 16.1584) -> (16.5463, 16.1584)
  line L464 (16.5463, 16.1584) -> (15.7663, 16.1584)
  line L465 (15.7663, 16.1584) -> (15.7663, 15.8884)
  arc A1352 (15.7663, 15.8884) -> (15.7706, 15.7849) centre (17.0031, 15.8884) ccw
  arc A1353 (15.7706, 15.7849) -> (15.7839, 15.6977) centre (16.4227, 15.8397) ccw
  arc A1354 (15.7839, 15.6977) -> (15.803, 15.6344) centre (16.2208, 15.7948) ccw
  arc A1355 (15.803, 15.6344) -> (15.8263, 15.6184) centre (15.8263, 15.6434) ccw
  arc A1356 (15.8536, 15.593) -> (15.8263, 15.6184) centre (15.8263, 15.591) ccw
  arc A1357 (15.8705, 15.3259) -> (15.8536, 15.593) centre (1.326, 14.5397) ccw
  arc A1358 (15.8826, 14.9789) -> (15.8705, 15.3259) centre (6.8073, 14.836) ccw
  arc A1359 (15.8863, 14.5084) -> (15.8826, 14.9789) centre (-13.9931, 14.5084) ccw
  arc A1360 (15.8831, 13.9247) -> (15.8863, 14.5084) centre (-38.2399, 14.5084) ccw
  arc A1361 (15.8702, 13.6173) -> (15.8831, 13.9247) centre (10.972, 13.9777) ccw
  arc A1362 (15.8484, 13.4355) -> (15.8702, 13.6173) centre (13.8738, 13.7641) ccw
  arc A1363 (15.8046, 13.3984) -> (15.8484, 13.4355) centre (15.8046, 13.4428) ccw
  arc A1364 (15.8046, 13.3984) -> (15.7683, 13.3831) centre (15.8046, 13.3477) ccw
  arc A1365 (15.7683, 13.3831) -> (15.7512, 13.3452) centre (15.8118, 13.3407) ccw
  arc A1366 (15.7512, 13.3452) -> (15.7553, 13.2705) centre (16.0424, 13.3237) ccw
  arc A1367 (15.7553, 13.2705) -> (15.7847, 13.1284) centre (19.1606, 13.9009) ccw
  arc A1368 (15.7847, 13.1284) -> (15.8393, 12.9436) centre (17.2967, 13.4744) ccw
  arc A1369 (15.8393, 12.9436) -> (15.9037, 12.8777) centre (15.9442, 12.9818) ccw
  arc A1370 (15.9037, 12.8777) -> (16.0071, 12.8727) centre (15.9629, 13.0297) ccw
  arc A1371 (16.0071, 12.8727) -> (16.2463, 12.9484) centre (14.9657, 16.5781) ccw
  arc A1372 (16.5095, 13.0326) -> (16.2463, 12.9484) centre (17.8052, 8.53) ccw
  arc A1373 (16.607, 13.0209) -> (16.5095, 13.0326) centre (16.5444, 12.9114) ccw
  arc A1374 (16.656, 12.9445) -> (16.607, 13.0209) centre (16.5585, 12.936) ccw
  arc A1375 (16.6663, 12.7084) -> (16.656, 12.9445) centre (13.9564, 12.7084) ccw
  line L466 (16.6663, 12.7084) -> (16.6663, 12.3784)
  line L467 (16.6663, 12.3784) -> (16.9363, 12.3784)
  arc A1376 (16.9363, 12.3784) -> (17.105, 12.3825) centre (16.9363, 15.8472) ccw
  arc A1377 (17.105, 12.3825) -> (17.1686, 12.4033) centre (17.0989, 12.5087) ccw
  arc A1378 (17.1686, 12.4033) -> (17.1984, 12.45) centre (17.1311, 12.4601) ccw
  arc A1379 (17.1984, 12.45) -> (17.2063, 12.5569) centre (16.4812, 12.5569) ccw
  arc A1380 (17.2101, 12.6652) -> (17.2063, 12.5569) centre (18.7233, 12.5569) ccw
  arc A1381 (17.2296, 12.7005) -> (17.2101, 12.6652) centre (17.2582, 12.6618) ccw
  arc A1382 (17.2683, 12.7074) -> (17.2296, 12.7005) centre (17.2559, 12.6648) ccw
  arc A1383 (17.366, 12.6747) -> (17.2683, 12.7074) centre (16.9127, 11.4822) ccw
  arc A1384 (17.366, 12.6747) -> (17.4306, 12.6549) centre (17.548, 13.1533) ccw
  arc A1385 (17.4306, 12.6549) -> (17.4924, 12.6457) centre (17.5172, 13.0223) ccw
  arc A1386 (17.4924, 12.6457) -> (17.5434, 12.6471) centre (17.5104, 12.919) ccw
  arc A1387 (17.5434, 12.6471) -> (17.5719, 12.6612) centre (17.5376, 12.6946) ccw
  arc A1388 (17.5719, 12.6612) -> (17.6157, 12.7367) centre (17.4442, 12.7858) ccw
  arc A1389 (17.6157, 12.7367) -> (17.7391, 13.1756) centre (-28.4691, 25.9297) ccw
  arc A1390 (17.7391, 13.1756) -> (17.8633, 13.6302) centre (-67.3933, 36.6733) ccw
  arc A1391 (17.8633, 13.6302) -> (17.851, 13.6724) centre (17.8226, 13.6412) ccw
  arc A1392 (17.851, 13.6724) -> (17.839, 13.6803) centre (17.8199, 13.6382) ccw
  arc A1393 (17.839, 13.6803) -> (17.7745, 13.7092) centre (13.5508, 4.2167) ccw
  arc A1394 (17.7745, 13.7092) -> (17.6986, 13.7423) centre (15.591, 8.802) ccw
  arc A1395 (17.6986, 13.7423) -> (17.6113, 13.779) centre (14.1093, 5.3288) ccw
  arc A1396 (17.6113, 13.779) -> (17.4737, 13.8336) centre (15.7455, 9.2768) ccw
  arc A1397 (17.4737, 13.8336) -> (17.42, 13.8424) centre (17.4252, 13.7058) ccw
  arc A1398 (17.42, 13.8424) -> (17.393, 13.8233) centre (17.4211, 13.8122) ccw
  arc A1399 (17.393, 13.8233) -> (17.3817, 13.7703) centre (17.5455, 13.7629) ccw
  arc A1400 (17.3749, 13.7158) -> (17.3817, 13.7703) centre (17.0296, 13.7863) ccw
  arc A1401 (17.3552, 13.6278) -> (17.3749, 13.7158) centre (15.0945, 14.1813) ccw
  arc A1402 (17.3286, 13.5278) -> (17.3552, 13.6278) centre (14.8004, 14.2533) ccw
  arc A1403 (17.298, 13.4284) -> (17.3286, 13.5278) centre (14.7598, 14.2649) ccw
  arc A1404 (17.2605, 13.3879) -> (17.298, 13.4284) centre (17.2347, 13.4492) ccw
  arc A1405 (17.2308, 13.4056) -> (17.2605, 13.3879) centre (17.2522, 13.4077) ccw
  arc A1406 (17.2188, 13.6327) -> (17.2308, 13.4056) centre (19.8551, 13.6583) ccw
  arc A1407 (17.2142, 14.2984) -> (17.2188, 13.6327) centre (138.1681, 14.808) ccw
  line L468 (17.2142, 14.2984) -> (17.2095, 15.4084)
  line L469 (17.2095, 15.4084) -> (17.3729, 15.2129)
  arc A1408 (17.3729, 15.2129) -> (17.4396, 15.138) centre (18.5687, 16.212) ccw
  arc A1409 (17.4396, 15.138) -> (17.5051, 15.0749) centre (18.2027, 15.8638) ccw
  arc A1410 (17.5051, 15.0749) -> (17.5623, 15.0281) centre (18.1361, 15.7885) ccw
  arc A1411 (17.5623, 15.0281) -> (17.5934, 15.0179) centre (17.5929, 15.0686) ccw
  arc A1412 (17.5934, 15.0179) -> (17.626, 15.0279) centre (17.5929, 15.0775) ccw
  arc A1413 (17.626, 15.0279) -> (17.6928, 15.0755) centre (16.8508, 16.1881) ccw
  arc A1414 (17.6928, 15.0755) -> (17.7704, 15.1386) centre (16.8282, 16.218) ccw
  arc A1415 (17.7704, 15.1386) -> (17.8516, 15.2132) centre (16.3796, 16.7319) ccw
  line L470 (17.8516, 15.2132) -> (18.0526, 15.408)
  line L471 (18.0526, 15.408) -> (17.9074, 15.0782)
  arc A1416 (17.8158, 14.8843) -> (17.9074, 15.0782) centre (14.2124, 16.7044) ccw
  arc A1417 (17.7513, 14.7968) -> (17.8158, 14.8843) centre (17.5251, 15.0311) ccw
  arc A1418 (17.6733, 14.7524) -> (17.7513, 14.7968) centre (17.6258, 14.9268) ccw
  arc A1419 (17.5465, 14.7299) -> (17.6733, 14.7524) centre (17.4855, 15.4415) ccw
  arc A1420 (17.5465, 14.7299) -> (17.4138, 14.7138) centre (17.7074, 12.8522) ccw
  arc A1421 (17.4138, 14.7138) -> (17.3656, 14.6871) centre (17.4264, 14.6342) ccw
  arc A1422 (17.3656, 14.6871) -> (17.3491, 14.6375) centre (17.4168, 14.6426) ccw
  arc A1423 (17.3491, 14.6375) -> (17.3637, 14.5199) centre (18.588, 14.7308) ccw
  arc A1424 (17.3637, 14.5199) -> (17.4102, 14.2964) centre (20.617, 15.0804) ccw
  arc A1425 (17.4102, 14.2964) -> (17.4621, 14.2224) centre (17.5309, 14.3259) ccw
  arc A1426 (17.4621, 14.2224) -> (17.5542, 14.1971) centre (17.5465, 14.3492) ccw
  arc A1427 (17.5542, 14.1971) -> (17.8191, 14.2168) centre (17.2694, 19.8161) ccw
  arc A1428 (18.0261, 14.2349) -> (17.8191, 14.2168) centre (18.7512, 4.7238) ccw
  arc A1429 (18.1119, 14.2319) -> (18.0261, 14.2349) centre (18.0555, 13.8486) ccw
  arc A1430 (18.1328, 14.2092) -> (18.1119, 14.2319) centre (18.1084, 14.2076) ccw
  arc A1431 (18.1197, 14.1726) -> (18.1328, 14.2092) centre (18.0843, 14.2059) ccw
  arc A1432 (18.1197, 14.1726) -> (18.0873, 14.1261) centre (18.2614, 14.0391) ccw
  arc A1433 (18.0873, 14.1261) -> (18.0843, 14.0867) centre (18.1341, 14.1027) ccw
  arc A1434 (18.0843, 14.0867) -> (18.1108, 14.0448) centre (18.1786, 14.117) ccw
  arc A1435 (18.1108, 14.0448) -> (18.1797, 13.9862) centre (18.7439, 14.7192) ccw
  line L472 (18.1797, 13.9862) -> (18.3163, 13.8811)
  line L473 (18.3163, 13.8811) -> (18.1213, 13.8797)
  line L474 (18.1213, 13.8797) -> (17.9263, 13.8784)
  line L475 (17.9263, 13.8784) -> (17.9263, 13.2205)
  arc A1436 (17.9263, 13.2205) -> (17.9389, 12.7201) centre (27.8537, 13.2205) ccw
  arc A1437 (17.9389, 12.7201) -> (18.0045, 12.541) centre (18.2608, 12.7364) ccw
  arc A1438 (18.0045, 12.541) -> (18.1518, 12.458) centre (18.1744, 12.6705) ccw
  arc A1439 (18.1518, 12.458) -> (18.5223, 12.4384) centre (18.5223, 15.9451) ccw
  arc A1440 (18.5223, 12.4384) -> (18.7777, 12.46) centre (18.5223, 13.9601) ccw
  arc A1441 (18.7777, 12.46) -> (18.9676, 12.5268) centre (18.6777, 13.0471) ccw
  arc A1442 (18.9676, 12.5268) -> (19.0838, 12.6343) centre (18.8041, 12.8203) ccw
  arc A1443 (19.0838, 12.6343) -> (19.1263, 12.7748) centre (18.8724, 12.7748) ccw
  arc A1444 (19.1323, 12.8138) -> (19.1263, 12.7748) centre (19.2551, 12.7748) ccw
  arc A1445 (19.1502, 12.8373) -> (19.1323, 12.8138) centre (19.1741, 12.8006) ccw
  arc A1446 (19.1795, 12.8446) -> (19.1502, 12.8373) centre (19.1756, 12.7983) ccw
  arc A1447 (19.2196, 12.8354) -> (19.1795, 12.8446) centre (19.1669, 12.6981) ccw
  arc A1448 (19.2196, 12.8354) -> (19.3311, 12.8281) centre (19.2871, 13.0112) ccw
  arc A1449 (19.3311, 12.8281) -> (19.5148, 12.8858) centre (19.0003, 14.2044) ccw
  arc A1450 (19.5148, 12.8858) -> (19.6856, 12.9649) centre (18.9611, 14.3051) ccw
  arc A1451 (19.6856, 12.9649) -> (19.7263, 13.0331) centre (19.6487, 13.0331) ccw
  arc A1452 (19.7263, 13.0331) -> (19.7082, 13.1388) centre (19.4085, 13.0331) ccw
  arc A1453 (19.7082, 13.1388) -> (19.596, 13.4473) centre (4.0737, 7.6255) ccw
  arc A1454 (19.596, 13.4473) -> (19.4773, 13.7547) centre (3.2662, 7.3227) ccw
  arc A1455 (19.4773, 13.7547) -> (19.4233, 13.841) centre (19.2159, 13.651) ccw
  arc A1456 (19.4233, 13.841) -> (19.3639, 13.8676) centre (19.3629, 13.7857) ccw
  arc A1457 (19.3639, 13.8676) -> (19.2521, 13.8582) centre (19.3568, 13.2785) ccw
  arc A1458 (19.2521, 13.8582) -> (19.1267, 13.8235) centre (19.3782, 13.1597) ccw
  arc A1459 (19.1267, 13.8235) -> (19.0168, 13.7676) centre (19.3295, 13.2883) ccw
  arc A1460 (19.0168, 13.7676) -> (18.9816, 13.7303) centre (19.0766, 13.6761) ccw
  arc A1461 (18.9816, 13.7303) -> (18.9703, 13.6834) centre (19.0566, 13.6874) ccw
  arc A1462 (18.9703, 13.6834) -> (18.9839, 13.6139) centre (19.2137, 13.6949) ccw
  arc A1463 (18.9839, 13.6139) -> (19.0297, 13.4948) centre (21.0926, 14.3567) ccw
  line L476 (19.0297, 13.4948) -> (19.1221, 13.2737)
  line L477 (19.1221, 13.2737) -> (18.9227, 13.3112)
  arc A1464 (18.9227, 13.3112) -> (18.8031, 13.3281) centre (18.6735, 11.9827) ccw
  arc A1465 (18.8031, 13.3281) -> (18.7477, 13.3151) centre (18.7946, 13.2401) ccw
  arc A1466 (18.7477, 13.3151) -> (18.7141, 13.2716) centre (18.7898, 13.2477) ccw
  arc A1467 (18.7141, 13.2716) -> (18.6863, 13.1635) centre (19.6978, 12.9612) ccw
  arc A1468 (18.6366, 12.9987) -> (18.6863, 13.1635) centre (17.7996, 13.3408) ccw
  arc A1469 (18.5825, 12.9896) -> (18.6366, 12.9987) centre (18.6067, 13.0109) ccw
  arc A1470 (18.5369, 13.0966) -> (18.5825, 12.9896) centre (18.7225, 13.1125) ccw
  arc A1471 (18.5263, 13.3457) -> (18.5369, 13.0966) centre (21.4581, 13.3457) ccw
  arc A1472 (18.5291, 13.5399) -> (18.5263, 13.3457) centre (25.2946, 13.3457) ccw
  arc A1473 (18.5418, 13.6283) -> (18.5291, 13.5399) centre (18.9194, 13.5287) ccw
  arc A1474 (18.5681, 13.6551) -> (18.5418, 13.6283) centre (18.5784, 13.6187) ccw
  arc A1475 (18.6058, 13.6471) -> (18.5681, 13.6551) centre (18.5794, 13.6152) ccw
  arc A1476 (18.6058, 13.6471) -> (18.655, 13.6273) centre (18.6611, 13.7137) ccw
  arc A1477 (18.655, 13.6273) -> (18.7102, 13.6382) centre (18.6625, 13.7345) ccw
  arc A1478 (18.7102, 13.6382) -> (18.7805, 13.686) centre (18.5724, 13.9166) ccw
  arc A1479 (18.7805, 13.686) -> (18.8817, 13.7836) centre (17.3721, 15.2467) ccw
  line L478 (18.8817, 13.7836) -> (19.078, 13.9862)
  line L479 (19.078, 13.9862) -> (18.8887, 14.1261)
  line L480 (18.8887, 14.1261) -> (18.6995, 14.266)
  line L481 (18.6995, 14.266) -> (18.8652, 14.3103)
  arc A1480 (18.9462, 14.3249) -> (18.8652, 14.3103) centre (18.9928, 13.8332) ccw
  arc A1481 (19.0158, 14.322) -> (18.9462, 14.3249) centre (18.9704, 14.0695) ccw
  arc A1482 (19.0771, 14.3011) -> (19.0158, 14.322) centre (18.9776, 14.1093) ccw
  arc A1483 (19.1332, 14.2622) -> (19.0771, 14.3011) centre (18.9545, 14.0647) ccw
  arc A1484 (19.1332, 14.2622) -> (19.1971, 14.2146) centre (19.4111, 14.5692) ccw
  arc A1485 (19.1971, 14.2146) -> (19.2496, 14.2006) centre (19.2476, 14.2983) ccw
  arc A1486 (19.2496, 14.2006) -> (19.313, 14.2145) centre (19.2462, 14.3676) ccw
  arc A1487 (19.313, 14.2145) -> (19.4257, 14.2681) centre (18.5575, 15.947) ccw
  arc A1488 (19.4257, 14.2681) -> (19.5471, 14.354) centre (19.1785, 14.7461) ccw
  arc A1489 (19.5471, 14.354) -> (19.5751, 14.4402) centre (19.4825, 14.4227) ccw
  arc A1490 (19.5751, 14.4402) -> (19.524, 14.5686) centre (19.2187, 14.3727) ccw
  arc A1491 (19.524, 14.5686) -> (19.3063, 14.8984) centre (6.7601, 6.3784) ccw
  line L482 (19.3063, 14.8984) -> (19.0634, 15.256)
  line L483 (19.0634, 15.256) -> (19.2716, 15.1332)
  line L484 (19.2716, 15.1332) -> (19.4798, 15.0104)
  line L485 (19.4798, 15.0104) -> (19.6106, 15.2669)
  arc A1492 (19.6106, 15.2669) -> (19.6722, 15.3955) centre (17.1141, 16.5405) ccw
  arc A1493 (19.6722, 15.3955) -> (19.6966, 15.474) centre (19.3544, 15.5377) ccw
  arc A1494 (19.6966, 15.474) -> (19.6923, 15.5217) centre (19.6102, 15.4901) ccw
  arc A1495 (19.6923, 15.5217) -> (19.6633, 15.5494) centre (19.6484, 15.5048) ccw
  arc A1496 (19.5366, 15.6219) -> (19.6633, 15.5494) centre (19.7805, 15.9011) ccw
  arc A1497 (19.3144, 15.8272) -> (19.5366, 15.6219) centre (23.0935, 19.6937) ccw
  arc A1498 (19.1036, 16.0446) -> (19.3144, 15.8272) centre (23.243, 19.8467) ccw
  arc A1499 (19.0345, 16.1639) -> (19.1036, 16.0446) centre (19.3386, 16.2604) ccw
  arc A1500 (19.0345, 16.1639) -> (19.001, 16.2208) centre (18.8934, 16.1192) ccw
  arc A1501 (19.001, 16.2208) -> (18.9468, 16.2558) centre (18.9028, 16.128) ccw
  arc A1502 (18.9468, 16.2558) -> (18.8572, 16.2736) centre (18.8363, 15.9348) ccw
  arc A1503 (18.8572, 16.2736) -> (18.7022, 16.2784) centre (18.7022, 13.7645) ccw
  line L486 (18.7022, 16.2784) -> (18.4063, 16.2784)
  line L487 (18.4063, 16.2784) -> (18.4063, 16.0684)
  arc A1504 (16.6599, 15.3974) -> (16.6663, 15.4684) centre (16.2689, 15.4684) ccw
  arc A1505 (16.6393, 15.3521) -> (16.6599, 15.3974) centre (16.56, 15.4156) ccw
  arc A1506 (16.6024, 15.327) -> (16.6393, 15.3521) centre (16.5796, 15.3999) ccw
  arc A1507 (16.5463, 15.3184) -> (16.6024, 15.327) centre (16.5463, 15.5067) ccw
  arc A1508 (16.4902, 15.327) -> (16.5463, 15.3184) centre (16.5463, 15.5067) ccw
  arc A1509 (16.4533, 15.3521) -> (16.4902, 15.327) centre (16.5129, 15.3999) ccw
  arc A1510 (16.4327, 15.3974) -> (16.4533, 15.3521) centre (16.5325, 15.4156) ccw
  arc A1511 (16.4263, 15.4684) -> (16.4327, 15.3974) centre (16.8237, 15.4684) ccw
  arc A1512 (16.4327, 15.5394) -> (16.4263, 15.4684) centre (16.8237, 15.4684) ccw
  arc A1513 (16.4533, 15.5846) -> (16.4327, 15.5394) centre (16.5325, 15.5212) ccw
  arc A1514 (16.4902, 15.6098) -> (16.4533, 15.5846) centre (16.5129, 15.5369) ccw
  arc A1515 (16.5463, 15.6184) -> (16.4902, 15.6098) centre (16.5463, 15.4301) ccw